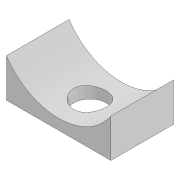
# Autodesk Inventor part: Tube_adaptor_2
Saved by Autodesk Inventor 2022 (Build 260153000, 153)
## iProperties
Created: 2022-06-09
Part Number: Tube_adaptor_2
Material: Generic
Document SubType Name: Modeling
Designer: dell
Density: 1 g/cm^3
Appearance: Default
Author: dell
Autodesk Inventor part; units mm, degrees
ref_plane "YZ Plane" through (0, 0, 0) normal (1, 0, 0) x (0, 1, 0)
ref_plane "XZ Plane" through (0, 0, 0) normal (0, 1, 0) x (-1, 0, 0)
ref_plane "XY Plane" through (0, 0, 0) normal (0, 0, 1) x (1, 0, 0)
sketch "Sketch1" plane through (0, 0, 0) normal (0, 0, 1) x (1, 0, 0)
  circle A0 centre (0, 0) radius 6
  line L0 (-5, 0) -> (5, 0)
  line L1 (5, 0) -> (5, -7)
  line L2 (5, -7) -> (-5, -7)
  line L3 (-5, -7) -> (-5, 0)
  point P0 (5, -3.3166)
  point P1 (-5, -3.3166)
  dimension "d0" = 12
  dimension "d1" = 1
  dimension "d2" = 5
  dimension "d3" = 5
  constraints: 8 end point, 2 parallel, 1 centre point, 1 coincident, 1 horizontal, 1 midpoint, 1 perpendicular
  measures "d0" diameter of A0
  measures "d1" distance edge to line of A0 L2
  measures "d2" distance from line of point (0, 0) L1
  measures "d3" distance from line of point (0, 0) L3
extrude "Extrusion1" add sketch "Sketch1" along normal blind 6 contours A0 L1 L2 L3
sketch "Sketch2" plane through (-5, -7, 0) normal (0, -1, 0) x (1, 0, 0)
  line L0 (0, 0) -> (10, 0) projected
  line L1 (10, 0) -> (10, 6) projected
  line L2 (0, 6) -> (10, 6) projected
  line L3 (0, 0) -> (0, 6) projected
  line L4 (0, 6) -> (10, 6) construction
  line L5 (10, 0) -> (0, 6) construction
  line L6 (0, 0) -> (10, 0) construction
  line L7 (10, 6) -> (0, 0) construction
  circle A0 centre (5, 3) radius 1.55
  point P0 (5, 0)
  dimension "d6" = 3.1
  constraints: 4 end point, 1 centre point, 1 midpoint
  measures "d6" diameter of A0
extrude "Extrusion2" cut sketch "Sketch2" along normal mid plane 6 contours A0
body "Solid1"
